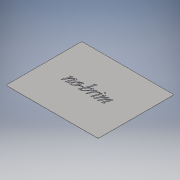
# Autodesk Inventor part: Lamiera logo no-brim
Saved by Autodesk Inventor 2018 (Build 220112000, 112)
## iProperties
Created: 2020-06-01
Part Number: Lamiera logo no-brim
Material: Generico
Document SubType Name: Lamiera
Designer: Francesco
Density: 1 g/cm^3
Sheet Metal Rule: Default_mm
Appearance: Acciaio - Lucido
Author: Francesco
Autodesk Inventor part; units mm, degrees
ref_plane "YZ Plane" through (0, 0, 0) normal (1, 0, 0) x (0, 1, 0)
ref_plane "XZ Plane" through (0, 0, 0) normal (0, 1, 0) x (-1, 0, 0)
ref_plane "XY Plane" through (0, 0, 0) normal (0, 0, 1) x (1, 0, 0)
sketch "Schizzo1" plane through (0, 0, 0) normal (0, 0, 1) x (1, 0, 0)
  line L0 (-335, 275.25) -> (335, 275.25)
  line L1 (335, 275.25) -> (335, -275.25)
  line L2 (335, -275.25) -> (-335, -275.25)
  line L3 (-335, -275.25) -> (-335, 275.25)
  line L4 (-335, 275.25) -> (335, -275.25) construction
  line L5 (335, 275.25) -> (-335, -275.25) construction
  point P0 (0, 0)
  dimension "d0" = 670
  dimension "d1" = 550.5
  measures "d0" distance of L1.end L2.end
  measures "d1" distance of L0.end L1.end
extrude "Piano1" add sketch "Schizzo1" along normal blind 1
fillet "Arrotondamento angolo1" radius 10 4 edges at (335, 275.25, 0.5) (-335, 275.25, 0.5) (335, -275.25, 0.5) (-335, -275.25, 0.5)
sketch "Schizzo2" plane through (0, 0, 1) normal (0, 0, 1) x (1, 0, 0)
  line L0 (-157.4575, 51.7567) -> (134.7822, 51.7567) construction
  line L1 (134.7822, 51.7567) -> (134.7822, -31.7703) construction
  line L2 (134.7822, -31.7703) -> (-157.4575, -31.7703) construction
  line L3 (-157.4575, -31.7703) -> (-157.4575, 51.7567) construction
  line L4 (-123.9933, -27.6417) -> (-122.9144, -29.5504)
  spline S0 degree 2 poles (-122.9144, -29.5504) (-131.2962, -35.5255) (-142.7484, -37.9321) knots 0 0 0 1 1 1
  spline S1 degree 2 poles (-142.7484, -37.9321) (-141.2547, -26.3969) (-129.1385, -2.9114) knots 0 0 0 1 1 1
  line L5 (-129.1385, -2.9114) -> (-124.6572, 5.7193)
  spline S2 degree 2 poles (-124.6572, 5.7193) (-122.3335, 10.2006) (-122.3335, 11.4455) knots 0 0 0 1 1 1
  spline S3 degree 2 poles (-122.3335, 11.4455) (-122.3335, 13.3542) (-123.8273, 13.3542) knots 0 0 0 1 1 1
  spline S4 degree 2 poles (-123.8273, 13.3542) (-126.0679, 13.3542) (-138.1011, 3.5616) (-143.8273, -2.8284) knots 0 0 0 1 2 2 2
  spline S5 degree 2 poles (-143.8273, -2.8284) (-155.6945, -16.1064) (-163.7443, -34.6956) knots 0 0 0 1 1 1
  spline S6 degree 2 poles (-163.7443, -34.6956) (-166.9808, -35.4425) (-172.9559, -38.0151) knots 0 0 0 1 1 1
  spline S7 degree 2 poles (-172.9559, -38.0151) (-166.5659, -24.9031) (-153.5368, 7.794) (-153.5368, 10.7816) knots 0 0 0 1 2 2 2
  spline S8 degree 2 poles (-153.5368, 10.7816) (-153.5368, 13.2712) (-155.5285, 13.2712) knots 0 0 0 1 1 1
  spline S9 degree 2 poles (-155.5285, 13.2712) (-156.6074, 13.2712) (-160.0928, 12.1923) knots 0 0 0 1 1 1
  spline S10 degree 2 poles (-160.0928, 12.1923) (-160.3418, 12.1094) (-160.8397, 12.0264) knots 0 0 0 1 1 1
  line L6 (-160.8397, 12.0264) -> (-161.2547, 14.1841)
  spline S11 degree 2 poles (-161.2547, 14.1841) (-151.4621, 17.0056) (-143.5783, 20.4911) knots 0 0 0 1 1 1
  line L7 (-143.5783, 20.4911) -> (-142.7484, 20.906)
  spline S12 degree 2 poles (-142.7484, 20.906) (-142.5825, 19.9932) (-142.5825, 19.6612) knots 0 0 0 1 1 1
  spline S13 degree 2 poles (-142.5825, 19.6612) (-142.5825, 13.4372) (-151.7111, -6.7288) knots 0 0 0 1 1 1
  line L8 (-151.7111, -6.7288) -> (-152.707, -8.8035)
  line L9 (-152.707, -8.8035) -> (-151.4621, -7.4757)
  spline S14 degree 2 poles (-151.4621, -7.4757) (-140.0928, 5.5533) (-120.7567, 20.5741) (-115.2796, 20.5741) knots 0 0 0 1 2 2 2
  spline S15 degree 2 poles (-115.2796, 20.5741) (-111.8771, 20.5741) (-111.8771, 17.0886) knots 0 0 0 1 1 1
  spline S16 degree 2 poles (-111.8771, 17.0886) (-111.8771, 13.4372) (-121.0057, -4.3222) knots 0 0 0 1 1 1
  spline S17 degree 2 poles (-121.0057, -4.3222) (-131.9601, -25.567) (-131.9601, -28.2226) knots 0 0 0 1 1 1
  spline S18 degree 2 poles (-131.9601, -28.2226) (-131.9601, -30.2143) (-130.0514, -30.2143) knots 0 0 0 1 1 1
  spline S19 degree 2 poles (-130.0514, -30.2143) (-127.9767, -30.2143) (-124.4082, -27.9736) knots 0 0 0 1 1 1
  line L10 (-124.4082, -27.9736) -> (-123.9933, -27.6417)
  spline S20 degree 2 poles (-64.4082, 13.6861) (-68.0597, 14.0181) (-70.5493, 14.0181) knots 0 0 0 1 1 1
  spline S21 degree 2 poles (-70.5493, 14.0181) (-88.8895, 14.0181) (-98.6821, -0.0068) knots 0 0 0 1 1 1
  spline S22 degree 2 poles (-98.6821, -0.0068) (-102.4995, -5.65) (-107.8107, -20.0068) (-107.8107, -24.9031) knots 0 0 0 1 2 2 2
  spline S23 degree 2 poles (-107.8107, -24.9031) (-107.8107, -28.3056) (-103.8273, -32.7039) (-100.7567, -32.7039) knots 0 0 0 1 2 2 2
  spline S24 degree 2 poles (-100.7567, -32.7039) (-93.4538, -32.7039) (-75.8605, -9.4674) (-75.8605, 0.2421) knots 0 0 0 1 2 2 2
  spline S25 degree 2 poles (-75.8605, 0.2421) (-75.8605, 2.3998) (-78.1841, 5.3874) (-79.7609, 5.3874) knots 0 0 0 1 2 2 2
  spline S26 degree 2 poles (-79.7609, 5.3874) (-85.3211, 5.3874) (-90.4663, -5.8159) knots 0 0 0 1 1 1
  spline S27 degree 2 poles (-90.4663, -5.8159) (-90.7982, -4.4052) (-90.7982, -3.3263) knots 0 0 0 1 1 1
  spline S28 degree 2 poles (-90.7982, -3.3263) (-90.7982, 0.989) (-80.0928, 10.4496) (-75.1966, 10.4496) knots 0 0 0 1 2 2 2
  spline S29 degree 2 poles (-75.1966, 10.4496) (-72.0431, 10.4496) (-67.5617, 5.2214) (-67.5617, 1.487) knots 0 0 0 1 2 2 2
  spline S30 degree 2 poles (-67.5617, 1.487) (-67.5617, -11.1272) (-83.6613, -25.235) knots 0 0 0 1 1 1
  spline S31 degree 2 poles (-83.6613, -25.235) (-97.5202, -37.5172) (-106.6489, -37.5172) knots 0 0 0 1 1 1
  spline S32 degree 2 poles (-106.6489, -37.5172) (-110.6323, -37.5172) (-115.8605, -31.7911) (-115.8605, -27.4757) knots 0 0 0 1 2 2 2
  spline S33 degree 2 poles (-115.8605, -27.4757) (-115.8605, -17.9321) (-102.5825, 2.8977) (-91.6281, 10.4496) knots 0 0 0 1 2 2 2
  spline S34 degree 2 poles (-91.6281, 10.4496) (-85.653, 14.516) (-71.5451, 19.8272) (-66.5659, 19.8272) knots 0 0 0 1 2 2 2
  spline S35 degree 2 poles (-66.5659, 19.8272) (-63.4953, 19.8272) (-63.4953, 17.0886) knots 0 0 0 1 1 1
  spline S36 degree 2 poles (-63.4953, 17.0886) (-63.4953, 16.0098) (-64.4082, 13.6861) knots 0 0 0 1 1 1
  line L11 (-64.5742, -5.318) -> (-55.0306, -5.318)
  line L12 (-55.0306, -5.318) -> (-52.292, -5.318)
  spline S37 degree 2 poles (-52.292, -5.318) (-46.7319, -5.318) (-42.9974, -3.4093) knots 0 0 0 1 1 1
  spline S38 degree 2 poles (-42.9974, -3.4093) (-42.9144, -3.3263) (-42.7484, -3.3263) knots 0 0 0 1 1 1
  line L13 (-42.7484, -3.3263) -> (-42.9144, -3.7413)
  line L14 (-42.9144, -3.7413) -> (-43.4123, -4.8201)
  spline S39 degree 2 poles (-43.4123, -4.8201) (-46.2339, -11.2931) (-55.2796, -11.2931) knots 0 0 0 1 1 1
  line L15 (-55.2796, -11.2931) -> (-58.5161, -11.2931)
  line L16 (-58.5161, -11.2931) -> (-62.0016, -11.2931)
  spline S40 degree 2 poles (-62.0016, -11.2931) (-64.4912, -11.2931) (-66.3169, -12.206) (-67.3128, -13.7828) knots 0 0 0 1 2 2 2
  line L17 (-67.3128, -13.7828) -> (-67.7277, -14.4467)
  line L18 (-67.7277, -14.4467) -> (-68.9725, -14.4467)
  line L19 (-68.9725, -14.4467) -> (-64.5742, -5.318)
  spline S41 degree 2 poles (-5.2381, 58.0845) (-6.0679, 47.628) (-24.3252, 4.2255) knots 0 0 0 1 1 1
  line L20 (-24.3252, 4.2255) -> (-25.57, 1.404)
  spline S42 degree 2 poles (-25.57, 1.404) (-18.0182, 9.6197) (-0.1758, 20.0762) (6.3802, 20.0762) knots 0 0 0 1 2 2 2
  spline S43 degree 2 poles (6.3802, 20.0762) (12.7702, 20.0762) (12.7702, 13.2712) knots 0 0 0 1 1 1
  spline S44 degree 2 poles (12.7702, 13.2712) (12.7702, 5.6363) (-1.1717, -14.7786) (-11.9601, -22.9944) knots 0 0 0 1 2 2 2
  spline S45 degree 2 poles (-11.9601, -22.9944) (-31.6281, -37.7662) (-49.9684, -37.7662) knots 0 0 0 1 1 1
  line L21 (-49.9684, -37.7662) -> (-49.0555, -35.5255)
  spline S46 degree 2 poles (-49.0555, -35.5255) (-35.9435, -5.318) (-16.7733, 43.5616) (-16.7733, 46.4662) knots 0 0 0 1 2 2 2
  spline S47 degree 2 poles (-16.7733, 46.4662) (-16.7733, 48.5409) (-19.263, 48.5409) knots 0 0 0 1 1 1
  spline S48 degree 2 poles (-19.263, 48.5409) (-20.8397, 48.5409) (-24.2422, 47.2961) knots 0 0 0 1 1 1
  line L22 (-24.2422, 47.2961) -> (-25.0721, 49.4538)
  spline S49 degree 2 poles (-25.0721, 49.4538) (-15.9435, 52.7733) (-5.2381, 58.0845) knots 0 0 0 1 1 1
  spline S50 degree 2 poles (-39.5119, -30.7952) (-37.6862, -31.0442) (-36.6904, -31.0442) knots 0 0 0 1 1 1
  spline S51 degree 2 poles (-36.6904, -31.0442) (-21.2547, -31.0442) (-9.1385, -15.5255) knots 0 0 0 1 1 1
  spline S52 degree 2 poles (-9.1385, -15.5255) (-4.2422, -9.2184) (2.2308, 4.9724) (2.2308, 9.3708) knots 0 0 0 1 2 2 2
  spline S53 degree 2 poles (2.2308, 9.3708) (2.2308, 14.267) (-2.3335, 14.267) knots 0 0 0 1 1 1
  spline S54 degree 2 poles (-2.3335, 14.267) (-10.3003, 14.267) (-32.7899, -13.0359) (-39.5119, -30.7952) knots 0 0 0 1 2 2 2
  line L23 (54.43, 19.8272) -> (51.9403, 12.8563)
  spline S55 degree 2 poles (51.9403, 12.8563) (49.2847, 13.4372) (47.293, 13.4372) knots 0 0 0 1 1 1
  spline S56 degree 2 poles (47.293, 13.4372) (39.1603, 13.4372) (29.9486, 0.989) knots 0 0 0 1 1 1
  spline S57 degree 2 poles (29.9486, 0.989) (25.6333, -4.9031) (19.4092, -18.845) (14.8449, -33.2018) knots 0 0 0 1 2 2 2
  line L24 (14.8449, -33.2018) -> (14.098, -35.5255)
  spline S58 degree 2 poles (14.098, -35.5255) (9.5337, -36.5213) (5.3843, -37.9321) knots 0 0 0 1 1 1
  line L25 (5.3843, -37.9321) -> (6.2142, -35.7745)
  line L26 (6.2142, -35.7745) -> (12.3553, -19.5089)
  spline S59 degree 2 poles (12.3553, -19.5089) (21.069, 4.0596) (21.069, 8.2089) knots 0 0 0 1 1 1
  spline S60 degree 2 poles (21.069, 8.2089) (21.069, 10.3666) (19.1603, 10.3666) knots 0 0 0 1 1 1
  spline S61 degree 2 poles (19.1603, 10.3666) (18.1644, 10.3666) (14.513, 8.5409) knots 0 0 0 1 1 1
  line L27 (14.513, 8.5409) -> (13.6001, 10.6986)
  spline S62 degree 2 poles (13.6001, 10.6986) (23.3096, 15.4289) (31.1105, 21.155) knots 0 0 0 1 1 1
  spline S63 degree 2 poles (31.1105, 21.155) (31.3594, 19.9102) (31.3594, 18.9143) knots 0 0 0 1 1 1
  spline S64 degree 2 poles (31.3594, 18.9143) (31.3594, 13.5202) (26.5462, 0.989) knots 0 0 0 1 1 1
  line L28 (26.5462, 0.989) -> (28.2059, 2.8977)
  spline S65 degree 2 poles (28.2059, 2.8977) (44.4715, 20.8231) (51.1935, 20.8231) knots 0 0 0 1 1 1
  spline S66 degree 2 poles (51.1935, 20.8231) (52.6872, 20.8231) (54.43, 19.8272) knots 0 0 0 1 1 1
  line L29 (70.4466, 21.8189) -> (70.4466, 21.072)
  spline S67 degree 2 poles (70.4466, 21.072) (70.4466, 14.516) (61.8159, -4.9031) knots 0 0 0 1 1 1
  line L30 (61.8159, -4.9031) -> (56.6706, -16.6043)
  spline S68 degree 2 poles (56.6706, -16.6043) (52.6042, -25.9819) (52.4383, -28.1396) knots 0 0 0 1 1 1
  spline S69 degree 2 poles (52.4383, -28.1396) (52.3553, -30.2973) (54.7619, -30.1313) knots 0 0 0 1 1 1
  spline S70 degree 2 poles (54.7619, -30.1313) (56.1727, -30.0483) (59.4092, -28.6375) knots 0 0 0 1 1 1
  line L31 (59.4092, -28.6375) -> (60.3221, -30.6292)
  spline S71 degree 2 poles (60.3221, -30.6292) (49.3677, -35.8574) (42.8117, -38.0981) knots 0 0 0 1 1 1
  spline S72 degree 2 poles (42.8117, -38.0981) (43.1437, -31.5421) (46.7121, -20.5047) (52.6042, -7.6417) knots 0 0 0 1 2 2 2
  spline S73 degree 2 poles (52.6042, -7.6417) (60.0731, 8.7899) (60.2391, 11.6114) knots 0 0 0 1 1 1
  spline S74 degree 2 poles (60.2391, 11.6114) (60.4051, 13.7691) (58.4134, 13.7691) knots 0 0 0 1 1 1
  spline S75 degree 2 poles (58.4134, 13.7691) (57.5005, 13.7691) (56.0897, 13.2712) knots 0 0 0 1 1 1
  line L32 (56.0897, 13.2712) -> (53.1852, 12.1923)
  spline S76 degree 2 poles (53.1852, 12.1923) (52.8532, 12.1094) (51.8574, 11.6944) knots 0 0 0 1 1 1
  line L33 (51.8574, 11.6944) -> (51.1105, 13.9351)
  line L34 (51.1105, 13.9351) -> (52.6042, 14.433)
  spline S77 degree 2 poles (52.6042, 14.433) (60.3221, 17.2546) (68.3719, 20.8231) knots 0 0 0 1 1 1
  line L35 (68.3719, 20.8231) -> (70.4466, 21.8189)
  spline S78 degree 2 poles (74.513, 39.6612) (77.7495, 39.6612) (77.7495, 36.4247) knots 0 0 0 1 1 1
  spline S79 degree 2 poles (77.7495, 36.4247) (77.7495, 34.599) (74.8449, 31.6944) (73.1022, 31.6944) knots 0 0 0 1 2 2 2
  spline S80 degree 2 poles (73.1022, 31.6944) (69.7827, 31.6944) (69.7827, 34.9309) knots 0 0 0 1 1 1
  spline S81 degree 2 poles (69.7827, 34.9309) (69.7827, 36.7567) (72.6872, 39.6612) (74.513, 39.6612) knots 0 0 0 1 2 2 2
  line L36 (136.5877, -27.3097) -> (137.7495, -29.1355)
  spline S82 degree 2 poles (137.7495, -29.1355) (130.3636, -34.4467) (120.1561, -37.7662) knots 0 0 0 1 1 1
  spline S83 degree 2 poles (120.1561, -37.7662) (121.235, -22.5794) (134.513, 4.4745) knots 0 0 0 1 1 1
  line L37 (134.513, 4.4745) -> (136.5047, 8.7899)
  spline S84 degree 2 poles (136.5047, 8.7899) (137.0856, 9.7857) (137.0856, 10.5326) knots 0 0 0 1 1 1
  spline S85 degree 2 poles (137.0856, 10.5326) (137.0856, 12.1923) (135.5918, 12.1923) knots 0 0 0 1 1 1
  spline S86 degree 2 poles (135.5918, 12.1923) (132.6042, 12.1923) (123.7246, 3.3127) knots 0 0 0 1 1 1
  spline S87 degree 2 poles (123.7246, 3.3127) (117.3345, -3.1603) (105.9652, -23.0774) (102.3968, -33.8657) knots 0 0 0 1 2 2 2
  spline S88 degree 2 poles (102.3968, -33.8657) (98.2474, -34.9446) (92.5213, -37.7662) knots 0 0 0 1 1 1
  line L38 (92.5213, -37.7662) -> (93.2681, -35.7745)
  line L39 (93.2681, -35.7745) -> (97.5005, -25.567)
  spline S89 degree 2 poles (97.5005, -25.567) (102.0648, -14.1977) (109.6167, 7.96) (109.6167, 10.3666) knots 0 0 0 1 2 2 2
  spline S90 degree 2 poles (109.6167, 10.3666) (109.6167, 12.3583) (107.708, 12.3583) knots 0 0 0 1 1 1
  spline S91 degree 2 poles (107.708, 12.3583) (105.3843, 12.3583) (94.347, 1.155) (89.6167, -6.1479) knots 0 0 0 1 2 2 2
  spline S92 degree 2 poles (89.6167, -6.1479) (81.4009, -18.845) (75.3428, -34.1977) knots 0 0 0 1 1 1
  spline S93 degree 2 poles (75.3428, -34.1977) (74.43, -34.5296) (74.264, -34.5296) knots 0 0 0 1 1 1
  line L40 (74.264, -34.5296) -> (70.5296, -35.8574)
  spline S94 degree 2 poles (70.5296, -35.8574) (68.2889, -36.6873) (65.9652, -37.6002) knots 0 0 0 1 1 1
  spline S95 degree 2 poles (65.9652, -37.6002) (67.625, -34.0317) (72.5213, -22.2475) knots 0 0 0 1 1 1
  line L41 (72.5213, -22.2475) -> (77.9984, -9.2184)
  spline S96 degree 2 poles (77.9984, -9.2184) (84.0565, 5.7193) (84.3055, 9.4538) knots 0 0 0 1 1 1
  spline S97 degree 2 poles (84.3055, 9.4538) (84.4715, 11.9434) (82.3138, 11.9434) knots 0 0 0 1 1 1
  spline S98 degree 2 poles (82.3138, 11.9434) (80.903, 11.9434) (78.0814, 10.6986) knots 0 0 0 1 1 1
  line L42 (78.0814, 10.6986) -> (77.2516, 12.9392)
  spline S99 degree 2 poles (77.2516, 12.9392) (83.3096, 15.2629) (92.8532, 21.155) knots 0 0 0 1 1 1
  line L43 (92.8532, 21.155) -> (94.43, 22.1509)
  spline S100 degree 2 poles (94.43, 22.1509) (94.596, 20.5741) (94.596, 19.4953) knots 0 0 0 1 1 1
  spline S101 degree 2 poles (94.596, 19.4953) (94.596, 13.5202) (87.376, -4.0732) knots 0 0 0 1 1 1
  spline S102 degree 2 poles (87.376, -4.0732) (106.7951, 20.6571) (117.4175, 20.6571) knots 0 0 0 1 1 1
  spline S103 degree 2 poles (117.4175, 20.6571) (120.5711, 20.6571) (120.5711, 17.3376) knots 0 0 0 1 1 1
  spline S104 degree 2 poles (120.5711, 17.3376) (120.5711, 12.2753) (113.5171, -4.9861) knots 0 0 0 1 1 1
  spline S105 degree 2 poles (113.5171, -4.9861) (121.5669, 5.5533) (140.3221, 20.7401) (145.3843, 20.7401) knots 0 0 0 1 2 2 2
  spline S106 degree 2 poles (145.3843, 20.7401) (148.2889, 20.7401) (148.2889, 17.8355) knots 0 0 0 1 1 1
  spline S107 degree 2 poles (148.2889, 17.8355) (148.2889, 15.7608) (142.9777, 4.4745) knots 0 0 0 1 1 1
  spline S108 degree 2 poles (142.9777, 4.4745) (130.1976, -22.9114) (130.1976, -27.3097) knots 0 0 0 1 1 1
  spline S109 degree 2 poles (130.1976, -27.3097) (130.1976, -29.2184) (132.0233, -29.2184) knots 0 0 0 1 1 1
  spline S110 degree 2 poles (132.0233, -29.2184) (133.3511, -29.2184) (136.5877, -27.3097) knots 0 0 0 1 1 1
  point P0 (0, 0)
  constraints: 2 other
extrude "Estrusione1" cut sketch "Schizzo2" against normal up to next
equation "\"d2\" = Spessore"
equation "\"RaggioPiega\" = Spessore"
equation "\"LarghezzaScaricoPiega\" = Spessore"
equation "\"ProfonditàScaricoPiega\" = 0.5 * Spessore"
equation "\"DimensioniScaricoAngolo\" = 4 * Spessore"
equation "\"ResiduoMinimo\" = 2 * Spessore"
equation "\"RaggioTransizione\" = RaggioPiega"
equation "\"Dimensione_raggio_Jacobi\" = RaggioPiega"
equation "\"DimensioneGioco\" = Spessore"
equation "\"Spessore\" = 1"
